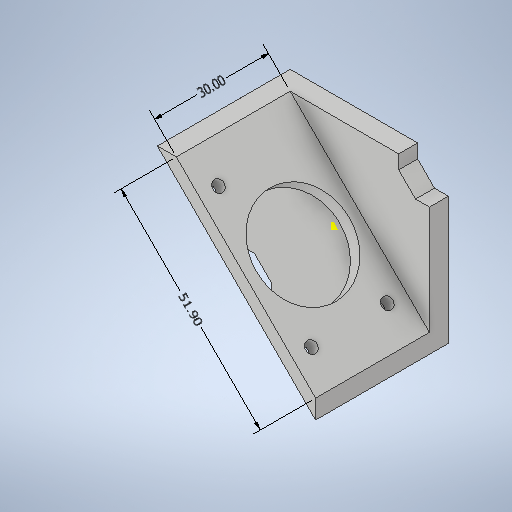
# Autodesk Inventor part: 可调底座
Saved by Autodesk Inventor 2025 (Build 290162000, 162)
## iProperties
Created: 2024-08-27
Part Number: 可调底座
Material: Generic
Document SubType Name: Sheet Metal
Designer: Administrator
Density: 1 g/cm^3
Sheet Metal Rule: 默认_mm
Appearance: Default
Author: Administrator
Autodesk Inventor part; units mm, degrees
ref_plane "YZ Plane" through (0, 0, 0) normal (1, 0, 0) x (0, 1, 0)
ref_plane "XZ Plane" through (0, 0, 0) normal (0, 1, 0) x (-1, 0, 0)
ref_plane "XY Plane" through (0, 0, 0) normal (0, 0, 1) x (1, 0, 0)
sketch "草图1" plane through (0, 0, 0) normal (0, 0, 1) x (1, 0, 0)
  line L0 (24.9, 0) -> (24.9, 16.8)
  line L1 (24.9, 0) -> (41.7, 0) construction
  line L2 (24.9, 16.8) -> (21.24, 16.8)
  line L3 (21.24, 16.8) -> (16.7994, 21.2406)
  line L4 (16.7994, 21.2406) -> (16.7994, 24.9006)
  line L5 (16.7994, 24.9006) -> (-0.0006, 24.9006)
  line L6 (24.9, 0) -> (24.9, -16.8)
  line L7 (24.9, -16.8) -> (21.24, -16.8)
  line L8 (21.24, -16.8) -> (16.7994, -21.2406)
  line L9 (16.7994, -21.2406) -> (16.7994, -24.9006)
  line L10 (16.7994, -24.9006) -> (-0.0006, -24.9006)
  line L11 (-0.0006, -24.9006) -> (-16.8006, -24.9006)
  line L12 (-16.8006, -24.9006) -> (-16.8006, -21.2406)
  line L13 (-16.8006, -21.2406) -> (-21.2413, -16.8)
  line L14 (-21.2413, -16.8) -> (-24.9013, -16.8)
  line L15 (-24.9013, -16.8) -> (-24.9013, 0)
  line L16 (-24.9013, 0) -> (-24.9013, 16.8)
  line L17 (-24.9013, 16.8) -> (-21.2413, 16.8)
  line L18 (-21.2413, 16.8) -> (-16.8006, 21.2406)
  line L19 (-16.8006, 21.2406) -> (-16.8006, 24.9006)
  line L20 (-16.8006, 24.9006) -> (-0.0006, 24.9006)
  point P0 (0, 0)
  constraints: 42 end point, 10 perpendicular, 4 point on line, 3 vertical, 2 parallel, 1 horizontal
extrude "拉伸1" add sketch "草图1" along normal blind 5
sketch "草图2" plane through (0, 0, 5) normal (0, 0, 1) x (1, 0, 0)
  point P0 (0, 0)
sketch "草图3" plane through (0, 0, 5) normal (0, 0, 1) x (1, 0, 0)
  line L0 (21.24, -16.8) -> (-16.8006, 21.2406)
  line L1 (-16.8006, 24.9006) -> (-16.8006, 21.2406) projected
  line L2 (-16.8006, 24.9006) -> (-11.8006, 24.9006)
  line L3 (16.7994, 24.9006) -> (-16.8006, 24.9006) projected
  line L4 (21.24, -16.8) -> (24.9, -16.8) projected
  line L5 (24.9, -16.8) -> (24.9, -11.8)
  line L6 (24.9, -16.8) -> (24.9, 16.8) projected
  line L7 (24.9, -11.8) -> (-11.8006, 24.9006)
  point P0 (0, 0)
  constraints: 8 end point, 2 point on line
extrude "拉伸2" add sketch "草图3" along normal blind 30
sketch "草图4" plane through (-11.8006, 24.9006, 5) normal (0.7071068, 0.7071068, 0) x (-0.7071068, 0.7071068, 0)
  line L0 (-51.9025, 0) -> (-51.9025, 30) projected
  line L1 (0, 0) -> (0, 30) projected
  line L2 (-51.9025, 30) -> (0, 0) construction
  line L3 (-51.9025, 30) -> (0, 30) projected
  line L4 (0, 30) -> (-51.9025, 0) construction
  point P0 (-25.9517, -5)
  point P1 (-25.9513, 15)
  constraints: 4 end point, 1 midpoint
hole "孔1" at (6.5497, 6.5503, 20) direction (-0.7071068, -0.7071068, 0) diameter 24.5 end through all
sketch "草图5" plane through (-11.8006, 24.9006, 5) normal (0.7071068, 0.7071068, 0) x (-0.7071068, 0.7071068, 0)
  line L0 (-51.9025, 0) -> (-51.9025, 30) projected
  line L1 (0, 0) -> (-51.9025, 0) projected
  line L2 (0, 0) -> (0, 30) projected
  line L3 (-12.9646, 7.4936) -> (-25.9513, 15) construction
  point P0 (-25.9517, -5)
  constraints: 5 other
hole "孔2" at (6.5497, 6.5503, 20) direction (-0.7071068, -0.7071068, 0) diameter 0.01 end through all
sketch "草图6" plane through (0, 0, 35) normal (0, 0, 1) x (1, 0, 0)
  line L0 (-11.8006, 24.9006) -> (-16.8006, 24.9006) projected
  line L1 (-16.8006, 24.9006) -> (-16.8006, 21.2406) projected
  line L2 (-16.8006, 24.9006) -> (-16.8006, 21.2406)
  line L3 (21.24, -16.8) -> (-16.8006, 21.2406) projected
  line L4 (-16.8006, 21.2406) -> (21.24, -16.8)
  line L5 (24.9, -16.8) -> (24.9, 16.8) projected
  line L6 (-16.8006, 24.9006) -> (24.9, -16.8)
  line L7 (24.9, -16.8) -> (21.24, -16.8)
  point P0 (0, 0)
  constraints: 8 end point, 1 collinear, 1 perpendicular, 1 vertical
extrude "拉伸3" cut sketch "草图6" against normal blind 30
sketch "草图7" plane through (-11.8006, 24.9006, 5) normal (0.7071068, 0.7071068, 0) x (-0.7071068, 0.7071068, 0)
  line L0 (-51.9025, 0) -> (-51.9025, 30) projected
  line L1 (0, 0) -> (0, 30) projected
  line L2 (-51.9025, 30) -> (0, 0)
  line L3 (-51.9025, 0) -> (0, 30)
  line L4 (-25.9513, 15) -> (-43.2669, 25.0085)
  line L5 (-25.9513, 15) -> (-7.1239, 25.8823)
  line L6 (-25.9513, 15) -> (-8.6357, 25.0085)
  line L7 (-25.9513, 15) -> (-41.7093, 5.8917)
  line L8 (-25.9513, 15) -> (-43.2669, 4.9915)
  point P0 (-25.9517, -5)
  constraints: 14 end point, 5 point on line, 3 coincident, 1 midpoint
hole "孔3" at (18.7937, -5.6937, 30.0085) at (18.7937, -5.6937, 9.9915) at (-5.6943, 18.7943, 30.0085) direction (-0.7071068, -0.7071068, 0) diameter 2.97 end through all
equation "\"d41\" = Thickness"
equation "\"BendRadius\" = Thickness"
equation "\"BendReliefWidth\" = Thickness"
equation "\"BendReliefDepth\" = 0.5 * Thickness"
equation "\"CornerReliefSize\" = 4 * Thickness"
equation "\"MinimumRemnant\" = 2 * Thickness"
equation "\"TransitionRadius\" = BendRadius"
equation "\"GapSize\" = Thickness"
equation "\"Thickness\" = 0.5"
